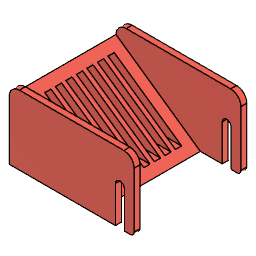
Cámara Oscura + Tolva (Autodesk Fusion 360 archive; units mm, degrees)
design "Tolva de Carga"
Autodesk Fusion 360 part; units mm, degrees
note: some values were not read from the file. Set by a fixed rule: which face or edge a step refers to.
sketch "Boceto1" plane through (0, 0, 0) normal (0, 1, 0) x (1, 0, 0)
  line L0 (0, 0) -> (50, 0)
  line L1 (0, 0) -> (0, -35)
  line L2 (0, -35) -> (50, 0)
  dimension "d1" = 50
  dimension "d2" = 35
  constraint coincident L0.start L1.start
  constraint horizontal L0
  constraint perpendicular L0 L1
  measures "d1" distance of L0.start L0.end
  measures "d2" distance of L0.start L1.end
extrude "Extruir1" add sketch "Boceto1" along normal blind 49 makes body 1
sketch "Boceto2" plane through (0, 0, 0) normal (0, -1, 0) x (1, 0, 0)
  line L0 (0, 35) -> (0, 0)
  line L1 (0, 0) -> (50, 0)
  line L2 (50, 0) -> (0, 35)
  line L3 (0, 35) -> (50, 35)
  line L4 (50, 35) -> (50, 0)
  line L5 (50, 0) -> (0, 0)
  line L6 (0, 0) -> (0, 35)
  line L7 (50, 0) -> (50, 6)
  line L8 (50, 6) -> (58, 6)
  line L9 (58, 6) -> (58, 35)
  line L10 (58, 35) -> (50, 35)
  line L11 (50, 35) -> (50, 6)
  dimension "d5" = 6
  dimension "d6" = 8
  constraint horizontal L3
  constraint vertical L4
  constraint horizontal L5
  constraint vertical L6
  constraint coincident L1.end L2.start
  constraint coincident L0.start L2.end
  constraint perpendicular L5 L7
  constraint horizontal L8
  constraint vertical L9
  constraint horizontal L10
  constraint vertical L11
  measures "d5" distance of L1.end L7.end
  measures "d6" distance of L7.end L8.end
extrude "Extruir2" add sketch "Boceto2" along normal blind 2 bodies 1
sketch "Boceto3" plane through (0, 49, 0) normal (0, 1, 0) x (-1, 0, 0)
  line L0 (0, 0) -> (0, 35)
  line L1 (0, 35) -> (-50, 0)
  line L2 (-50, 0) -> (0, 0)
  line L3 (0, 0) -> (-50, 0)
  line L4 (-50, 0) -> (-50, 35)
  line L5 (-50, 35) -> (0, 35)
  line L6 (0, 35) -> (0, 0)
  line L7 (-58, 35) -> (-50, 35)
  line L8 (-50, 35) -> (-50, 6)
  line L9 (-50, 6) -> (-58, 6)
  line L10 (-58, 6) -> (-58, 35)
  dimension "d13" = 8
  constraint horizontal L3
  constraint vertical L4
  constraint horizontal L5
  constraint vertical L6
  constraint coincident L0.start L2.end
  constraint horizontal L7
  constraint vertical L8
  constraint horizontal L9
  constraint vertical L10
  constraint coincident L4 L8.end
  measures "d13" distance of L8.end L9.end
extrude "Extruir3" add sketch "Boceto3" along normal blind 2 bodies 1
sketch "Boceto4" plane through (0, -2, 0) normal (0, -1, 0) x (1, 0, 0)
  line L0 (50, 0) -> (50, 6)
  line L1 (50, 6) -> (58, 6)
  line L2 (58, 6) -> (58, 35)
  line L3 (58, 35) -> (0, 35)
  line L4 (0, 35) -> (0, 0)
  line L5 (0, 0) -> (50, 0)
  line L6 (50, 6) -> (56, 6)
  line L7 (56, 6) -> (52, 6)
  line L8 (52, 6) -> (52, 26)
  line L9 (52, 26) -> (56, 26)
  line L10 (56, 26) -> (56, 6)
  dimension "d11" = 4
  dimension "d12" = 20
  constraint coincident L0.end L1.start
  constraint coincident L1 L6.end
  constraint horizontal L7
  constraint vertical L8
  constraint horizontal L9
  constraint vertical L10
  measures "d11" distance of L6.end L7.end
  measures "d12" distance of L6.end L9.end
sketch "Boceto5" plane through (0, 49, 0) normal (0, -1, 0) x (1, 0, 0)
  line L0 (0, 35) -> (50, 0)
  line L1 (50, 0) -> (50, 6)
  line L2 (50, 6) -> (58, 6)
  line L3 (58, 6) -> (58, 35)
  line L4 (58, 35) -> (0, 35)
extrude "Extruir4" cut sketch "Boceto4" against normal blind 56 contours L1 L6 L7 L8 L9 L10 bodies 1
move_face "CarasDesfase1" offset 5 2 faces at (38.6667, 49.6667, 35) (19.3333, -0.6667, 35) on bodies 1
copy_body "Cuerpo - > Comp.1" bodies 1 removing the originals makes body 2 in component "Tolva"
fillet "Empalme2" radius 5 4 edges at (58, 50, 40) (58, -1, 40) (0, 50, 40) (0, -1, 40) on bodies 2 in component "Tolva"
sketch "Boceto6" plane through (50, 0, 0) normal (1, 0, 0) x (0, 1, 0)
  line L0 (-2, 6) -> (-2, 0)
  line L1 (-2, 0) -> (0, 0)
  line L2 (0, 0) -> (0, 6)
  line L3 (0, 35) -> (5, 35)
  line L4 (5, 35) -> (5, 32)
  line L5 (5, 32) -> (8, 32)
  line L6 (8, 32) -> (8, 9)
  line L7 (8, 9) -> (5, 9)
  line L8 (5, 9) -> (5, 32)
  line L9 (13.1429, 32) -> (13.1429, 9)
  line L10 (10.1429, 32) -> (13.1429, 32)
  line L11 (10.1429, 9) -> (10.1429, 32)
  line L12 (13.1429, 9) -> (10.1429, 9)
  line L13 (18.2857, 32) -> (18.2857, 9)
  line L14 (15.2857, 32) -> (18.2857, 32)
  line L15 (15.2857, 9) -> (15.2857, 32)
  line L16 (18.2857, 9) -> (15.2857, 9)
  line L17 (23.4286, 32) -> (23.4286, 9)
  line L18 (20.4286, 32) -> (23.4286, 32)
  line L19 (20.4286, 9) -> (20.4286, 32)
  line L20 (23.4286, 9) -> (20.4286, 9)
  line L21 (28.5714, 32) -> (28.5714, 9)
  line L22 (25.5714, 32) -> (28.5714, 32)
  line L23 (25.5714, 9) -> (25.5714, 32)
  line L24 (28.5714, 9) -> (25.5714, 9)
  line L25 (33.7143, 32) -> (33.7143, 9)
  line L26 (30.7143, 32) -> (33.7143, 32)
  line L27 (30.7143, 9) -> (30.7143, 32)
  line L28 (33.7143, 9) -> (30.7143, 9)
  line L29 (38.8571, 32) -> (38.8571, 9)
  line L30 (35.8571, 32) -> (38.8571, 32)
  line L31 (35.8571, 9) -> (35.8571, 32)
  line L32 (38.8571, 9) -> (35.8571, 9)
  line L33 (44, 32) -> (44, 9)
  line L34 (41, 32) -> (44, 32)
  line L35 (41, 9) -> (41, 32)
  line L36 (44, 9) -> (41, 9)
  line L37 (0, 6) -> (-2, 6)
  dimension "d21" = 3
  dimension "d22" = 23
  dimension "d31" = 36
  dimension "d32" = 0
  constraint horizontal L3
  constraint perpendicular L3 L4
  constraint horizontal L5
  constraint vertical L6
  constraint horizontal L7
  constraint vertical L8
  measures "d21" distance of L4.end L5.end
  measures "d22" distance of L4.end L7.end
extrude "Extruir1'" cut sketch "Boceto6" against normal blind 72 contours L5 L6 L7 L8 | L9 L10 L11 L12 | L13 L14 L15 L16 | L17 L18 L19 L20 | L21 L22 L23 L24 | L25 L26 L27 L28 | L29 L30 L31 L32 | L33 L34 L35 L36 bodies 2 in component "Tolva"
move_face "CarasDesfase2" offset -0.1 2 faces at (35.6666, 49, 24) (35.6666, 0, 24) on bodies 2 in component "Tolva"
extrude "Extruir2'" cut 1 faces at (16.6667, 32.7, 0) along direction (0, 0, 1) blind 5 on bodies 2 bodies 2 in component "Tolva"
extrude "Extruir3'" cut 1 faces at (14.2857, 16.3, 5) along direction (0, 0, 1) blind 1.15 on bodies 2 bodies 2 in component "Tolva"
move_face "CarasDesfase4" offset 1 2 faces at (19, -2, 24.05) (19, 51, 24.05) on bodies 2 in component "Tolva"
move_face "CarasDesfase5" offset 3 2 faces at (58, 51.0333, 25.3334) (58, -1.0667, 15.6667) on bodies 2 in component "Tolva"
extrude "Extruir4'" cut 2 faces at (51.3333, -2.0333, 6) (50.6667, 50.0667, 6) along direction (0, 0, -1) up to surface end surface through (50, 49, 6.15) normal (0, 0, -1) offset 0 on bodies 2 bodies 2 in component "Tolva"
fillet "Empalme5" radius 2 6 edges at (52, -1.55, 26) (56, -1.55, 26) (52, 50.55, 26) (56, 50.55, 26) (61, -1.55, 6) (61, 50.55, 6) on bodies 2 in component "Tolva"
move_face "CarasDesfase6" offset -0.15 10 faces at (52, -1.0667, 18.0503) (55.5722, -1.0667, 25.2365) (54.0001, -1.0667, 26) (52.0091, -1.0667, 24.1905) (56, -1.0667, 18.0003) (55.6292, 50.0667, 25.1603) (53.9999, 50.0667, 26) (52.4278, 50.0667, 25.2365) (52, 51.0333, 18.0503) (56, 50.0667, 18.0003) on bodies 2 in component "Tolva"
component "Tolva" placed x (1, 0, 0) y (0, 1, 0) z (0, 0, 1) at (0, 0, 0)
named bodies: "Tolva"

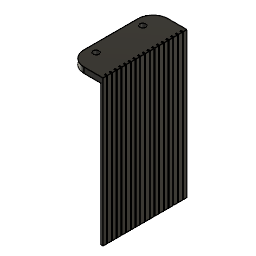
design "Cortina Lamas TPU"
Autodesk Fusion 360 part; units mm, degrees
sketch "Boceto1" plane through (0, 0, 0) normal (0, 0, 1) x (1, 0, 0)
  circle A0 centre (0, 0) radius 1.575
  line L0 (0, 0) -> (12.5, 0)
  line L1 (12.5, 0) -> (12.5, 10)
  line L2 (12.5, 0) -> (12.5, -25)
  line L3 (12.5, 10) -> (-4.5, 10)
  line L4 (-4.5, 10) -> (-4.5, -35)
  line L5 (-4.5, -35) -> (12.5, -35)
  line L6 (12.5, -35) -> (12.5, 10)
  line L7 (12.5, -25) -> (0, -25)
  circle A1 centre (0, -25) radius 1.575
  line L8 (12.5, 10) -> (13.7, 10)
  line L9 (13.7, 10) -> (13.7, 8)
  line L10 (13.7, 8) -> (12.5, 8)
  line L11 (12.5, 8) -> (12.5, 10)
  line L12 (13.7, 5.4706) -> (12.5, 5.4706)
  line L13 (13.7, 7.4706) -> (13.7, 5.4706)
  line L14 (12.5, 7.4706) -> (13.7, 7.4706)
  line L15 (12.5, 5.4706) -> (12.5, 7.4706)
  line L16 (13.7, 2.9412) -> (12.5, 2.9412)
  line L17 (13.7, 4.9412) -> (13.7, 2.9412)
  line L18 (12.5, 4.9412) -> (13.7, 4.9412)
  line L19 (12.5, 2.9412) -> (12.5, 4.9412)
  line L20 (13.7, 0.4118) -> (12.5, 0.4118)
  line L21 (13.7, 2.4118) -> (13.7, 0.4118)
  line L22 (12.5, 2.4118) -> (13.7, 2.4118)
  line L23 (12.5, 0.4118) -> (12.5, 2.4118)
  line L24 (13.7, -2.1176) -> (12.5, -2.1176)
  line L25 (13.7, -0.1176) -> (13.7, -2.1176)
  line L26 (12.5, -0.1176) -> (13.7, -0.1176)
  line L27 (12.5, -2.1176) -> (12.5, -0.1176)
  line L28 (13.7, -4.6471) -> (12.5, -4.6471)
  line L29 (13.7, -2.6471) -> (13.7, -4.6471)
  line L30 (12.5, -2.6471) -> (13.7, -2.6471)
  line L31 (12.5, -4.6471) -> (12.5, -2.6471)
  line L32 (13.7, -7.1765) -> (12.5, -7.1765)
  line L33 (13.7, -5.1765) -> (13.7, -7.1765)
  line L34 (12.5, -5.1765) -> (13.7, -5.1765)
  line L35 (12.5, -7.1765) -> (12.5, -5.1765)
  line L36 (13.7, -9.7059) -> (12.5, -9.7059)
  line L37 (13.7, -7.7059) -> (13.7, -9.7059)
  line L38 (12.5, -7.7059) -> (13.7, -7.7059)
  line L39 (12.5, -9.7059) -> (12.5, -7.7059)
  line L40 (13.7, -12.2353) -> (12.5, -12.2353)
  line L41 (13.7, -10.2353) -> (13.7, -12.2353)
  line L42 (12.5, -10.2353) -> (13.7, -10.2353)
  line L43 (12.5, -12.2353) -> (12.5, -10.2353)
  line L44 (13.7, -14.7647) -> (12.5, -14.7647)
  line L45 (13.7, -12.7647) -> (13.7, -14.7647)
  line L46 (12.5, -12.7647) -> (13.7, -12.7647)
  line L47 (12.5, -14.7647) -> (12.5, -12.7647)
  line L48 (13.7, -17.2941) -> (12.5, -17.2941)
  line L49 (13.7, -15.2941) -> (13.7, -17.2941)
  line L50 (12.5, -15.2941) -> (13.7, -15.2941)
  line L51 (12.5, -17.2941) -> (12.5, -15.2941)
  line L52 (13.7, -19.8235) -> (12.5, -19.8235)
  line L53 (13.7, -17.8235) -> (13.7, -19.8235)
  line L54 (12.5, -17.8235) -> (13.7, -17.8235)
  line L55 (12.5, -19.8235) -> (12.5, -17.8235)
  line L56 (13.7, -22.3529) -> (12.5, -22.3529)
  line L57 (13.7, -20.3529) -> (13.7, -22.3529)
  line L58 (12.5, -20.3529) -> (13.7, -20.3529)
  line L59 (12.5, -22.3529) -> (12.5, -20.3529)
  line L60 (13.7, -24.8824) -> (12.5, -24.8824)
  line L61 (13.7, -22.8824) -> (13.7, -24.8824)
  line L62 (12.5, -22.8824) -> (13.7, -22.8824)
  line L63 (12.5, -24.8824) -> (12.5, -22.8824)
  line L64 (13.7, -27.4118) -> (12.5, -27.4118)
  line L65 (13.7, -25.4118) -> (13.7, -27.4118)
  line L66 (12.5, -25.4118) -> (13.7, -25.4118)
  line L67 (12.5, -27.4118) -> (12.5, -25.4118)
  line L68 (13.7, -29.9412) -> (12.5, -29.9412)
  line L69 (13.7, -27.9412) -> (13.7, -29.9412)
  line L70 (12.5, -27.9412) -> (13.7, -27.9412)
  line L71 (12.5, -29.9412) -> (12.5, -27.9412)
  line L72 (13.7, -32.4706) -> (12.5, -32.4706)
  line L73 (13.7, -30.4706) -> (13.7, -32.4706)
  line L74 (12.5, -30.4706) -> (13.7, -30.4706)
  line L75 (12.5, -32.4706) -> (12.5, -30.4706)
  line L76 (13.7, -35) -> (12.5, -35)
  line L77 (13.7, -33) -> (13.7, -35)
  line L78 (12.5, -33) -> (13.7, -33)
  line L79 (12.5, -35) -> (12.5, -33)
  dimension "d1" = 3.15
  dimension "d2" = 12.5
  dimension "d3" = 10
  dimension "d4" = 25
  dimension "d5" = 17
  dimension "d6" = 45
  dimension "d7" = 12.5
  dimension "d8" = 3.15
  dimension "d9" = 1.2
  dimension "d10" = 2
  dimension "d13" = 0
  dimension "d14" = -43
  constraint coincident A0.centre L0.start
  constraint horizontal L0
  constraint perpendicular L0 L1
  constraint perpendicular L0 L2
  constraint horizontal L3
  constraint vertical L4
  constraint horizontal L5
  constraint vertical L6
  constraint perpendicular L6 L7
  constraint coincident L7.end A1.centre
  constraint horizontal L8
  constraint vertical L9
  constraint horizontal L10
  constraint vertical L11
  measures "d1" diameter of A0
  measures "d2" distance of A0.centre L0.end
  measures "d3" distance of L0.end L1.end
  measures "d4" distance of L0.end L2.end
  measures "d5" distance of L1.end L3.end
  measures "d6" distance of L1.end L5.end
  measures "d7" distance of L2.end L7.end
  measures "d8" diameter of A1
  measures "d9" distance of L1.end L8.end
  measures "d10" distance of L1.end L10.end
extrude "Extruir1" add sketch "Boceto1" along normal blind 3 makes body 1
copy_body "Cuerpo - > Comp.1" bodies 1 removing the originals makes body 2 in component "Cortina de Lamas"
extrude "Extruir1'" add sketch "Boceto1" against normal blind 75 contours L1 L6 L20 L21 L22 L23 | L2 L6 L24 L25 L26 L27 | L1 L6 L16 L17 L18 L19 | L2 L6 L28 L29 L30 L31 | L1 L6 L12 L13 L14 L15 | L2 L6 L32 L33 L34 L35 | L1 L6 L8 L9 L10 L11 | L2 L6 L36 L37 L38 L39 | L2 L6 L40 L41 L42 L43 | L6 L76 L77 L78 L79 | L2 L6 L44 L45 L46 L47 | L6 L72 L73 L74 L75 | L2 L6 L48 L49 L50 L51 | L6 L68 L69 L70 L71 | L2 L6 L52 L53 L54 L55 | L6 L64 L65 L66 L67 | L2 L6 L56 L57 L58 L59 | L2 L6 L60 L61 L62 L63 bodies 2 in component "Cortina de Lamas"
fillet "Empalme1" radius 8 2 edges at (-4.5, 10, 1.5) (-4.5, -35, 1.5) on bodies 2 in component "Cortina de Lamas"
component "Cortina de Lamas" placed x (1, 0, 0) y (0, 1, 0) z (0, 0, 1) at (0, 0, 0)
named bodies: "Cortina de Lamas"
